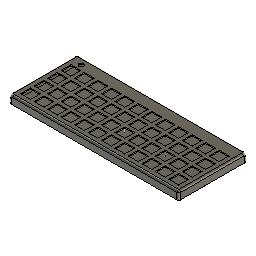
liteboard (Autodesk Fusion 360 design; units mm, degrees)
part number: 2026-04-12-12-30-01-683
Autodesk Fusion 360 part; units mm, degrees
(part 1 of 18)
sketch "草图2" plane through (0, 0, 0) normal (0, 0, 1) x (1, 0, 0)
  line L0 (4.2648, 0.88) -> (3.8878, 1.2675)
  line L1 (-10.3353, 1.2675) -> (0.4381, 1.2675)
  line L2 (0.0611, 0.88) -> (-0.1551, 0.3845)
  line L3 (0.4381, 1.2675) -> (0.0611, 0.88)
  line L4 (222.6289, -88.1864) -> (-10.3353, -88.1864)
  line L5 (-10.3353, -88.1864) -> (-10.3353, 1.2675)
  line L6 (222.6289, 1.2675) -> (222.6289, -88.1864)
  line L7 (4.5085, -0.1553) -> (4.481, 0.3845)
  line L8 (0.3176, -1.0941) -> (0.7811, -1.3723)
  line L9 (4.481, 0.3845) -> (4.2648, 0.88)
  line L10 (-0.1826, -0.1553) -> (-0.018, -0.6703)
  line L11 (3.8878, 1.2675) -> (222.6289, 1.2675)
  line L12 (4.0083, -1.0941) -> (4.3439, -0.6703)
  line L13 (3.0129, -1.4692) -> (3.5448, -1.3723)
  line L14 (4.3439, -0.6703) -> (4.5085, -0.1553)
  line L15 (0.7811, -1.3723) -> (1.3129, -1.4692)
  line L16 (-0.018, -0.6703) -> (0.3176, -1.0941)
  line L17 (3.5448, -1.3723) -> (4.0083, -1.0941)
  line L18 (-0.1551, 0.3845) -> (-0.1826, -0.1553)
  line L19 (1.3129, -1.4692) -> (3.0129, -1.4692)
  line L20 (-4.3556, -1.7588) -> (-4.8371, -1.663)
  line L21 (-5.9994, -3.4026) -> (-5.7267, -3.8108)
  line L22 (-3.6747, -3.4026) -> (-3.5789, -2.9211)
  line L23 (-3.9474, -2.0315) -> (-4.3556, -1.7588)
  line L24 (-4.8371, -4.1793) -> (-4.3556, -4.0835)
  line L25 (-5.7267, -3.8108) -> (-5.3185, -4.0835)
  line L26 (-4.8371, -1.663) -> (-5.3185, -1.7588)
  line L27 (-3.6747, -2.4397) -> (-3.9474, -2.0315)
  line L28 (-4.3556, -4.0835) -> (-3.9474, -3.8108)
  line L29 (-5.3185, -4.0835) -> (-4.8371, -4.1793)
  line L30 (-5.9994, -2.4397) -> (-6.0952, -2.9211)
  line L31 (-3.9474, -3.8108) -> (-3.6747, -3.4026)
  line L32 (-6.0952, -2.9211) -> (-5.9994, -3.4026)
  line L33 (-5.7267, -2.0315) -> (-5.9994, -2.4397)
  line L34 (-5.3185, -1.7588) -> (-5.7267, -2.0315)
  line L35 (-3.5789, -2.9211) -> (-3.6747, -2.4397)
  line L36 (-5.7267, -7.1115) -> (-5.9994, -7.5197)
  line L37 (-5.9994, -8.4826) -> (-5.7267, -8.8908)
  line L38 (-5.9994, -7.5197) -> (-6.0952, -8.0011)
  line L39 (-6.0952, -8.0011) -> (-5.9994, -8.4826)
  line L40 (-3.6747, -7.5197) -> (-3.9474, -7.1115)
  line L41 (-5.3185, -9.1635) -> (-4.8371, -9.2593)
  line L42 (-3.9474, -8.8908) -> (-3.6747, -8.4826)
  line L43 (-4.8371, -9.2593) -> (-4.3556, -9.1635)
  line L44 (-3.9474, -7.1115) -> (-4.3556, -6.8388)
  line L45 (-4.3556, -6.8388) -> (-4.8371, -6.743)
  line L46 (-4.8371, -6.743) -> (-5.3185, -6.8388)
  line L47 (-5.7267, -8.8908) -> (-5.3185, -9.1635)
  line L48 (-3.6747, -8.4826) -> (-3.5789, -8.0011)
  line L49 (-4.3556, -9.1635) -> (-3.9474, -8.8908)
  line L50 (-5.3185, -6.8388) -> (-5.7267, -7.1115)
  line L51 (-3.5789, -8.0011) -> (-3.6747, -7.5197)
  line L52 (2.8261, -21.8809) -> (3.418, -21.4267)
  line L53 (-1.3638, -20.1454) -> (-1.0782, -20.8347)
  line L54 (-1.0782, -17.9766) -> (-1.3638, -18.6659)
  line L55 (-0.0321, -21.8809) -> (0.6573, -22.1664)
  line L56 (4.1578, -18.6659) -> (3.8722, -17.9766)
  line L57 (2.8261, -16.9304) -> (2.1367, -16.6449)
  line L58 (-1.4611, -19.4056) -> (-1.3638, -20.1454)
  line L59 (3.8722, -17.9766) -> (3.418, -17.3846)
  line L60 (0.6573, -16.6449) -> (-0.0321, -16.9304)
  line L61 (2.1367, -16.6449) -> (1.397, -16.5475)
  line L62 (1.397, -16.5475) -> (0.6573, -16.6449)
  line L63 (3.418, -17.3846) -> (2.8261, -16.9304)
  line L64 (0.6573, -22.1664) -> (1.397, -22.2638)
  line L65 (3.8722, -20.8347) -> (4.1578, -20.1454)
  line L66 (-0.624, -21.4267) -> (-0.0321, -21.8809)
  line L67 (-0.624, -17.3846) -> (-1.0782, -17.9766)
  line L68 (1.397, -22.2638) -> (2.1367, -22.1664)
  line L69 (4.1578, -20.1454) -> (4.2551, -19.4056)
  line L70 (-0.0321, -16.9304) -> (-0.624, -17.3846)
  line L71 (4.2551, -19.4056) -> (4.1578, -18.6659)
  line L72 (2.1367, -22.1664) -> (2.8261, -21.8809)
  line L73 (3.418, -21.4267) -> (3.8722, -20.8347)
  line L74 (-1.0782, -20.8347) -> (-0.624, -21.4267)
  line L75 (-1.3638, -18.6659) -> (-1.4611, -19.4056)
  line L76 (-1.4611, -76.5812) -> (-1.3638, -77.3209)
  line L77 (0.6573, -73.8204) -> (-0.0321, -74.1059)
  line L78 (-1.0782, -75.1521) -> (-1.3638, -75.8414)
  line L79 (3.418, -74.5601) -> (2.8261, -74.1059)
  line L80 (0.6573, -79.3419) -> (1.397, -79.4393)
  line L81 (-0.0321, -79.0564) -> (0.6573, -79.3419)
  line L82 (3.8722, -75.1521) -> (3.418, -74.5601)
  line L83 (-0.624, -78.6022) -> (-0.0321, -79.0564)
  line L84 (3.418, -78.6022) -> (3.8722, -78.0102)
  line L85 (4.1578, -77.3209) -> (4.2551, -76.5812)
  line L86 (-1.3638, -75.8414) -> (-1.4611, -76.5812)
  line L87 (2.8261, -79.0564) -> (3.418, -78.6022)
  line L88 (2.1367, -73.8204) -> (1.397, -73.723)
  line L89 (1.397, -73.723) -> (0.6573, -73.8204)
  line L90 (1.397, -79.4393) -> (2.1367, -79.3419)
  line L91 (2.1367, -79.3419) -> (2.8261, -79.0564)
  line L92 (4.2551, -76.5812) -> (4.1578, -75.8414)
  line L93 (2.8261, -74.1059) -> (2.1367, -73.8204)
  line L94 (-0.624, -74.5601) -> (-1.0782, -75.1521)
  line L95 (-0.0321, -74.1059) -> (-0.624, -74.5601)
  line L96 (4.1578, -75.8414) -> (3.8722, -75.1521)
  line L97 (3.8722, -78.0102) -> (4.1578, -77.3209)
  line L98 (-1.3638, -77.3209) -> (-1.0782, -78.0102)
  line L99 (-1.0782, -78.0102) -> (-0.624, -78.6022)
  line L100 (-0.0321, -35.9805) -> (-0.624, -36.4347)
  line L101 (-0.624, -40.4767) -> (-0.0321, -40.9309)
  line L102 (2.1367, -35.6949) -> (1.397, -35.5975)
  line L103 (3.8722, -37.0266) -> (3.418, -36.4347)
  line L104 (4.1578, -39.1954) -> (4.2551, -38.4557)
  line L105 (-0.624, -36.4347) -> (-1.0782, -37.0266)
  line L106 (1.397, -41.3138) -> (2.1367, -41.2164)
  line L107 (-1.0782, -37.0266) -> (-1.3638, -37.7159)
  line L108 (3.8722, -39.8847) -> (4.1578, -39.1954)
  line L109 (-1.3638, -37.7159) -> (-1.4611, -38.4557)
  line L110 (1.397, -35.5975) -> (0.6573, -35.6949)
  line L111 (-1.3638, -39.1954) -> (-1.0782, -39.8847)
  line L112 (-1.4611, -38.4557) -> (-1.3638, -39.1954)
  line L113 (2.8261, -40.9309) -> (3.418, -40.4767)
  line L114 (-1.0782, -39.8847) -> (-0.624, -40.4767)
  line L115 (0.6573, -35.6949) -> (-0.0321, -35.9805)
  line L116 (4.2551, -38.4557) -> (4.1578, -37.7159)
  line L117 (3.418, -40.4767) -> (3.8722, -39.8847)
  line L118 (3.418, -36.4347) -> (2.8261, -35.9805)
  line L119 (2.1367, -41.2164) -> (2.8261, -40.9309)
  line L120 (2.8261, -35.9805) -> (2.1367, -35.6949)
  line L121 (4.1578, -37.7159) -> (3.8722, -37.0266)
  line L122 (-0.0321, -40.9309) -> (0.6573, -41.2164)
  line L123 (0.6573, -41.2164) -> (1.397, -41.3138)
  line L124 (-0.624, -55.4974) -> (-1.0782, -56.0893)
  line L125 (0.6573, -54.7577) -> (-0.0321, -55.0432)
  line L126 (2.8261, -59.9936) -> (3.418, -59.5394)
  line L127 (2.1367, -54.7577) -> (1.397, -54.6603)
  line L128 (3.418, -59.5394) -> (3.8722, -58.9475)
  line L129 (3.8722, -58.9475) -> (4.1578, -58.2582)
  line L130 (-1.3638, -56.7787) -> (-1.4611, -57.5184)
  line L131 (4.1578, -58.2582) -> (4.2551, -57.5184)
  line L132 (-0.0321, -55.0432) -> (-0.624, -55.4974)
  line L133 (4.1578, -56.7787) -> (3.8722, -56.0893)
  line L134 (-1.4611, -57.5184) -> (-1.3638, -58.2582)
  line L135 (-0.624, -59.5394) -> (-0.0321, -59.9936)
  line L136 (-1.0782, -56.0893) -> (-1.3638, -56.7787)
  line L137 (0.6573, -60.2792) -> (1.397, -60.3766)
  line L138 (1.397, -60.3766) -> (2.1367, -60.2792)
  line L139 (-1.3638, -58.2582) -> (-1.0782, -58.9475)
  line L140 (1.397, -54.6603) -> (0.6573, -54.7577)
  line L141 (3.418, -55.4974) -> (2.8261, -55.0432)
  line L142 (2.1367, -60.2792) -> (2.8261, -59.9936)
  line L143 (-0.0321, -59.9936) -> (0.6573, -60.2792)
  line L144 (4.2551, -57.5184) -> (4.1578, -56.7787)
  line L145 (3.8722, -56.0893) -> (3.418, -55.4974)
  line L146 (-1.0782, -58.9475) -> (-0.624, -59.5394)
  line L147 (2.8261, -55.0432) -> (2.1367, -54.7577)
  line L148 (175.0892, -23.1507) -> (175.1842, -23.6313)
  line L149 (200.443, -3.4264) -> (200.5548, -3.1425)
  line L150 (195.6981, -2.3541) -> (195.408, -2.2378)
  line L151 (206.2125, -2.532) -> (206.1424, -2.2351)
  line L152 (19.9512, -10.5182) -> (19.879, -10.5602)
  line L153 (172.2522, -5.3569) -> (167.1323, -5.3569)
  line L154 (1.3129, -12.4692) -> (2.985, -12.4692)
  line L155 (190.9024, 0.21) -> (190.8125, 0.6041)
  line L156 (172.2256, -3.3861) -> (172.2242, -3.418)
  line L157 (9.181, -1.759) -> (8.7706, -2.0343)
  line L158 (195.408, -2.2378) -> (195.0968, -2.2673)
  line L159 (167.1323, -5.3569) -> (166.9467, -5.3938)
  line L160 (215.5423, -1.3966) -> (215.5423, -11.302)
  line L161 (196.5703, -6.8777) -> (194.9024, -6.8777)
  line L162 (10.1501, -1.7611) -> (9.6657, -1.663)
  line L163 (173.5966, -1.369) -> (173.3141, -1.4382)
  line L164 (2.985, -12.4692) -> (3.1779, -12.6621)
  line L165 (176.3444, -21.8935) -> (175.864, -21.99)
  line L166 (215.6027, -11.9249) -> (215.8415, -12.1417)
  line L167 (8.7706, -2.0343) -> (8.4979, -2.4465)
  line L168 (190.9024, -0.5069) -> (190.9024, 0.21)
  line L169 (197.593, 0.2231) -> (191.8334, 0.2231)
  line L170 (201.9182, -1.8376) -> (202.224, -1.9247)
  line L171 (156.1344, -61.7447) -> (156.4058, -62.1522)
  line L172 (198.2393, 0.2231) -> (198.1398, 0.2231)
  line L173 (0.7971, -12.3782) -> (1.3129, -12.4692)
  line L174 (194.8338, -3.3523) -> (195.0969, -3.521)
  line L175 (10.8239, -8.4863) -> (164.9732, -8.4863)
  line L176 (156.4056, -24.0392) -> (156.8122, -24.3125)
  line L177 (180.5338, -0.9789) -> (180.7794, -1.2929)
  line L178 (167.3333, -6.3272) -> (189.3463, -6.3272)
  line L179 (189.3011, -6.8777) -> (167.1355, -6.8777)
  line L180 (201.5865, -1.3167) -> (201.688, -1.6181)
  line L181 (172.9618, -2.1747) -> (173.0851, -2.4381)
  line L182 (4.0055, -41.3139) -> (3.7341, -41.7214)
  line L183 (3.6389, -42.2017) -> (3.7341, -42.6819)
  line L184 (164.2644, -9.5479) -> (18.415, -9.5479)
  line L185 (175.3144, -1.5898) -> (175.5226, -1.8185)
  line L186 (197.8695, -1.6165) -> (198.0055, -1.3392)
  line L187 (10.5503, -8.8932) -> (10.8239, -8.4863)
  line L188 (182.2626, 0.21) -> (182.1727, 0.6041)
  line L189 (201.168, -0.6121) -> (202.1153, -0.6121)
  line L190 (202.224, -1.9247) -> (203.1744, -2.8751)
  line L191 (202.8355, -0.9556) -> (202.6463, -0.7323)
  line L192 (4.0074, -22.262) -> (3.7349, -22.6694)
  line L193 (195.9027, -2.5903) -> (195.6981, -2.3541)
  line L194 (10.1419, -6.8377) -> (9.6608, -6.743)
  line L195 (176.3475, -0.7849) -> (176.0783, -0.6326)
  line L196 (172.2299, -3.3545) -> (172.2256, -3.3861)
  line L197 (156.4058, -60.3767) -> (156.1344, -60.7842)
  line L198 (199.2895, -0.5484) -> (199.3507, -0.1912)
  line L199 (156.0392, -61.2644) -> (156.1344, -61.7447)
  line L200 (216.1544, -12.2202) -> (216.4673, -12.1417)
  line L201 (0.3435, -12.1163) -> (0.7971, -12.3782)
  line L202 (190.7902, -3.3527) -> (194.8338, -3.3523)
  line L203 (190.8739, -3.5643) -> (190.7902, -3.3527)
  line L204 (4.8954, -21.8935) -> (4.4148, -21.9896)
  line L205 (198.1922, -0.9586) -> (198.3525, -0.832)
  line L206 (201.637, -1.0027) -> (201.5865, -1.3167)
  line L207 (172.2313, -5.2888) -> (172.2522, -5.3569)
  line L208 (202.6463, -0.7323) -> (202.3795, -0.6121)
  line L209 (8.5005, -8.4821) -> (8.7726, -8.89)
  line L210 (198.7028, -0.925) -> (199.0496, -0.8201)
  line L211 (194.2339, -79.8483) -> (194.1393, -80.3294)
  line L212 (10.5503, -7.1091) -> (10.1419, -6.8377)
  line L213 (205.9467, -3.063) -> (206.1424, -2.8289)
  line L214 (18.2294, -9.5848) -> (18.072, -9.69)
  line L215 (190.8695, -5.1322) -> (190.9024, -4.8901)
  line L216 (166.9498, -6.9146) -> (166.7925, -7.0198)
  line L217 (182.1751, -0.9789) -> (182.2626, -0.59)
  line L218 (199.8039, -2.3916) -> (199.52, -2.5034)
  line L219 (216.7666, -11.302) -> (216.7666, -1.143)
  line L220 (202.9101, -1.2386) -> (202.8355, -0.9556)
  line L221 (205.3623, -1.8958) -> (205.0973, -2.0469)
  line L222 (180.5363, 0.6041) -> (180.4463, 0.21)
  line L223 (205.3623, -3.1682) -> (205.667, -3.1846)
  line L224 (190.5605, 0.92) -> (190.1964, 1.0954)
  line L225 (203.3317, -2.9802) -> (203.5174, -3.0171)
  line L226 (178.803, -0.8218) -> (178.6173, -0.7849)
  line L227 (199.52, -2.5034) -> (199.3163, -2.7304)
  line L228 (3.521, -12.8042) -> (16.129, -12.8042)
  line L229 (205.0973, -3.0171) -> (205.3623, -3.1682)
  line L230 (9.6608, -9.2593) -> (10.1419, -9.1646)
  line L231 (6.0579, -22.6665) -> (5.7844, -22.2598)
  line L232 (194.3243, -4.9814) -> (194.0618, -4.9249)
  line L233 (215.5423, -11.302) -> (215.4944, -11.621)
  line L234 (15.9281, -11.8339) -> (4.2428, -11.8339)
  line L235 (178.9604, -0.927) -> (178.803, -0.8218)
  line L236 (205.667, -1.8794) -> (205.3623, -1.8958)
  line L237 (189.0861, 0.21) -> (189.0861, -0.59)
  line L238 (9.2008, -4.0913) -> (9.6871, -4.179)
  line L239 (0.7971, -9.5438) -> (0.3435, -9.8057)
  line L240 (8.7726, -7.1123) -> (8.5005, -7.5202)
  line L241 (164.7723, -7.516) -> (10.8239, -7.516)
  line L242 (173.8815, -1.4273) -> (173.5966, -1.369)
  line L243 (8.7726, -8.89) -> (9.18, -9.1629)
  line L244 (216.5873, -0.7102) -> (215.4443, 0.4328)
  line L245 (189.3463, -6.3272) -> (189.2636, -6.5975)
  line L246 (205.0973, -2.0469) -> (203.7184, -2.0469)
  line L247 (197.6227, -1.8022) -> (197.8695, -1.6165)
  line L248 (194.6816, -5.3671) -> (194.5428, -5.1373)
  line L249 (4.4148, -21.9896) -> (4.0074, -22.262)
  line L250 (166.7925, -7.0198) -> (164.2644, -9.5479)
  line L251 (165.3162, -8.3442) -> (167.3333, -6.3272)
  line L252 (175.8118, -1.9279) -> (174.3183, -1.9279)
  line L253 (173.3141, -1.4382) -> (173.0884, -1.6216)
  line L254 (199.0496, -0.8201) -> (199.2895, -0.5484)
  line L255 (15.9233, -3.3705) -> (15.9425, -3.3693)
  line L256 (199.2357, -3.0246) -> (198.4743, -3.786)
  line L257 (19.8151, -10.6139) -> (7.7625, -22.6665)
  line L258 (181.5565, 1.0954) -> (181.1524, 1.0954)
  line L259 (4.5116, -10.7923) -> (4.3529, -10.2689)
  line L260 (180.4463, -0.59) -> (180.5338, -0.9789)
  line L261 (198.001, -1.0303) -> (198.1922, -0.9586)
  line L262 (200.5276, -2.8386) -> (200.3673, -2.5791)
  line L263 (190.8125, 0.6041) -> (190.5605, 0.92)
  line L264 (164.9732, -8.4863) -> (165.1589, -8.4494)
  line L265 (156.8122, -41.0408) -> (156.4058, -41.3139)
  line L266 (202.3795, -0.6121) -> (214.7579, -0.6121)
  line L267 (181.9295, -1.2929) -> (182.1751, -0.9789)
  line L268 (15.9041, -3.3709) -> (15.9233, -3.3705)
  line L269 (10.8381, -3.3709) -> (15.9041, -3.3709)
  line L270 (200.9144, 0.6121) -> (200.6801, 0.5655)
  line L271 (198.1618, -6.6507) -> (197.9434, -6.6507)
  line L272 (8.4979, -2.4465) -> (8.405, -2.9318)
  line L273 (175.5226, -1.8185) -> (175.8118, -1.9279)
  line L274 (193.7985, -4.9771) -> (193.5774, -5.1294)
  line L275 (181.1524, 1.0954) -> (180.7882, 0.92)
  line L276 (4.4119, -24.3125) -> (4.4119, -41.0408)
  line L277 (198.3322, -4.129) -> (198.3322, -6.0986)
  line L278 (197.6871, -6.4844) -> (197.3834, -6.4506)
  line L279 (3.6389, -23.1501) -> (3.7337, -23.6309)
  line L280 (215.8415, -12.1417) -> (216.1544, -12.2202)
  line L281 (189.1761, 0.6041) -> (189.0861, 0.21)
  line L282 (176.8251, -21.9878) -> (176.3444, -21.8935)
  line L283 (3.7349, -22.6694) -> (3.6389, -23.1501)
  line L284 (189.7922, 1.0954) -> (189.4281, 0.92)
  line L285 (9.6657, -1.663) -> (9.181, -1.759)
  line L286 (177.5102, -60.7842) -> (177.2389, -60.3767)
  line L287 (-0.1723, -10.6991) -> (-0.1723, -11.2229)
  line L288 (175.864, -21.99) -> (175.457, -22.2627)
  line L289 (190.1964, 1.0954) -> (189.7922, 1.0954)
  line L290 (171.9053, -13.3122) -> (185.5007, -13.3122)
  line L291 (189.1736, -0.9789) -> (189.4193, -1.2929)
  line L292 (215.0114, 0.6121) -> (200.9144, 0.6121)
  line L293 (158.4602, -60.7842) -> (158.1888, -60.3767)
  line L294 (216.8145, -11.621) -> (216.7666, -11.302)
  line L295 (195.8825, -60.1036) -> (195.8825, -43.3625)
  line L296 (194.2345, -42.6819) -> (194.5059, -43.0894)
  line L297 (201.3539, -9.7544) -> (201.0692, -9.8528)
  line L298 (200.2237, -9.1925) -> (199.9543, -9.3449)
  line L299 (177.2389, -41.3139) -> (176.8325, -41.0408)
  line L300 (209.4715, -9.0376) -> (209.6395, -9.2629)
  line L301 (175.8664, -81.4897) -> (176.3474, -81.5853)
  line L302 (205.1665, -11.5952) -> (204.8563, -11.7579)
  line L303 (175.1845, -60.7842) -> (175.0892, -61.2644)
  line L304 (209.9181, -10.4074) -> (210.2759, -10.3948)
  line L305 (203.0941, -11.1739) -> (203.07, -10.8729)
  line L306 (199.3025, -4.33) -> (199.9218, -3.7107)
  line L307 (194.2345, -61.7447) -> (194.5059, -62.1522)
  line L308 (202.915, -10.6139) -> (202.6612, -10.4504)
  line L309 (202.3612, -10.4164) -> (202.0772, -10.5189)
  line L310 (201.7756, -6.3295) -> (201.8474, -6.6507)
  line L311 (199.4729, -6.6507) -> (199.451, -6.3551)
  line L312 (199.9218, -3.7107) -> (200.216, -3.6301)
  line L313 (167.9834, -17.2341) -> (171.9053, -13.3122)
  line L314 (196.6555, -61.2644) -> (196.5603, -60.7842)
  line L315 (175.8622, -79.1663) -> (175.4553, -79.4399)
  line L316 (199.1561, -8.4813) -> (198.9102, -8.5383)
  line L317 (196.5608, -79.8483) -> (196.2894, -79.4399)
  line L318 (156.407, -22.2627) -> (156.1349, -22.6702)
  line L319 (163.5579, -16.4059) -> (163.3723, -16.4428)
  line L320 (163.2149, -16.548) -> (157.7751, -21.9878)
  line L321 (201.0073, -9.5495) -> (200.8146, -9.3074)
  line L322 (200.5329, -9.1791) -> (200.2237, -9.1925)
  line L323 (200.8146, -9.3074) -> (200.5329, -9.1791)
  line L324 (194.9123, -62.4253) -> (194.9123, -79.1663)
  line L325 (201.8474, -6.6507) -> (199.4729, -6.6507)
  line L326 (207.5885, -14.8215) -> (207.8381, -14.6519)
  line L327 (199.9543, -9.3449) -> (199.8121, -9.3449)
  line L328 (177.5102, -61.7447) -> (177.6055, -61.2644)
  line L329 (157.2943, -21.8935) -> (156.814, -21.99)
  line L330 (156.1342, -23.6313) -> (156.4056, -24.0392)
  line L331 (156.814, -21.99) -> (156.407, -22.2627)
  line L332 (156.1349, -22.6702) -> (156.0392, -23.1507)
  line L333 (158.5555, -80.3294) -> (158.4608, -79.8483)
  line L334 (158.1862, -81.2176) -> (158.459, -80.8102)
  line L335 (199.8121, -9.3449) -> (199.8414, -9.0942)
  line L336 (207.1491, -12.8136) -> (206.802, -12.8325)
  line L337 (199.3025, -6.0986) -> (199.3025, -4.33)
  line L338 (195.8825, -62.4253) -> (196.2889, -62.1522)
  line L339 (206.7888, -14.5552) -> (207.0032, -14.7675)
  line L340 (177.5102, -41.7214) -> (177.2389, -41.3139)
  line L341 (209.4835, -8.063) -> (209.6394, -8.263)
  line L342 (158.1894, -79.4399) -> (157.7825, -79.1663)
  line L343 (196.5591, -80.8102) -> (196.6555, -80.3294)
  line L344 (194.9123, -41.0408) -> (194.5059, -41.3139)
  line L345 (205.9605, -12.1223) -> (205.808, -11.807)
  line L346 (198.9102, -8.5383) -> (198.8429, -8.2682)
  line L347 (204.8563, -11.7579) -> (204.3641, -11.7579)
  line L348 (176.8325, -41.0408) -> (176.8325, -24.3125)
  line L349 (205.5162, -11.6133) -> (205.1665, -11.5952)
  line L350 (207.4581, -12.9728) -> (207.1491, -12.8136)
  line L351 (206.2819, -12.1114) -> (205.9605, -12.1223)
  line L352 (196.6555, -42.2017) -> (196.5603, -41.7214)
  line L353 (209.6059, -10.232) -> (209.9181, -10.4074)
  line L354 (212.2314, -10.4073) -> (212.5433, -10.2319)
  line L355 (199.7749, -8.8507) -> (199.6222, -8.6497)
  line L356 (177.2394, -79.4399) -> (176.8325, -79.1663)
  line L357 (157.7783, -81.4897) -> (158.1862, -81.2176)
  line L358 (194.9123, -79.1663) -> (194.5053, -79.4399)
  line L359 (196.2894, -79.4399) -> (195.8825, -79.1663)
  line L360 (195.8825, -41.0408) -> (195.8825, -24.3125)
  line L361 (209.4304, -9.9199) -> (209.6059, -10.232)
  line L362 (158.459, -80.8102) -> (158.5555, -80.3294)
  line L363 (156.8164, -81.4897) -> (157.2973, -81.5853)
  line L364 (194.9123, -43.3625) -> (194.9123, -60.1036)
  line L365 (196.5499, -22.647) -> (204.6418, -14.5552)
  line L366 (199.4054, -8.5203) -> (199.1561, -8.4813)
  line L367 (194.9123, -60.1036) -> (194.5059, -60.3767)
  line L368 (199.8414, -9.0942) -> (199.7749, -8.8507)
  line L369 (176.8283, -81.4897) -> (177.2362, -81.2176)
  line L370 (199.6222, -8.6497) -> (199.4054, -8.5203)
  line L371 (196.5603, -60.7842) -> (196.2889, -60.3767)
  line L372 (196.5653, -23.6196) -> (196.6554, -23.1318)
  line L373 (194.9123, -24.3125) -> (194.9123, -41.0408)
  line L374 (212.6779, -8.4885) -> (212.5099, -8.2631)
  line L375 (202.056, -10.2184) -> (201.9041, -9.9582)
  line L376 (157.7751, -21.9878) -> (157.2943, -21.8935)
  line L377 (175.8622, -43.3625) -> (175.8622, -60.1036)
  line L378 (167.4394, -16.4059) -> (163.5579, -16.4059)
  line L379 (199.451, -6.3551) -> (199.3025, -6.0986)
  line L380 (156.0392, -23.1507) -> (156.1342, -23.6313)
  line L381 (156.0392, -42.2017) -> (156.1344, -42.6819)
  line L382 (196.2889, -62.1522) -> (196.5603, -61.7447)
  line L383 (156.4058, -41.3139) -> (156.1344, -41.7214)
  line L384 (204.6418, -14.5552) -> (206.7888, -14.5552)
  line L385 (194.1393, -80.3294) -> (194.2357, -80.8102)
  line L386 (175.0892, -42.2017) -> (175.1845, -42.6819)
  line L387 (175.1845, -42.6819) -> (175.4558, -43.0894)
  line L388 (175.4558, -43.0894) -> (175.8622, -43.3625)
  line L389 (175.4558, -41.3139) -> (175.1845, -41.7214)
  line L390 (176.8325, -62.4253) -> (177.2389, -62.1522)
  line L391 (194.5059, -62.1522) -> (194.9123, -62.4253)
  line L392 (194.2315, -23.6245) -> (194.5031, -24.0366)
  line L393 (204.3489, -11.4872) -> (204.2266, -11.2452)
  line L394 (212.7375, -8.7631) -> (212.6779, -8.4885)
  line L395 (196.2862, -81.2176) -> (196.5591, -80.8102)
  line L396 (205.808, -11.807) -> (205.5162, -11.6133)
  line L397 (175.1856, -80.8102) -> (175.4585, -81.2176)
  line L398 (204.3641, -11.7579) -> (204.3489, -11.4872)
  line L399 (204.2266, -11.2452) -> (204.0177, -11.0724)
  line L400 (175.8622, -41.0408) -> (175.4558, -41.3139)
  line L401 (198.4239, -7.9208) -> (198.4014, -7.7372)
  line L402 (201.6528, -9.7922) -> (201.3539, -9.7544)
  line L403 (195.8825, -43.3625) -> (196.2889, -43.0894)
  line L404 (196.6554, -23.1318) -> (196.5499, -22.647)
  line L405 (194.5059, -41.3139) -> (194.2345, -41.7214)
  line L406 (212.5099, -8.2631) -> (212.6658, -8.0631)
  line L407 (157.7825, -62.4253) -> (158.1888, -62.1522)
  line L408 (158.4602, -61.7447) -> (158.5555, -61.2644)
  line L409 (208.0035, -14.0879) -> (207.8851, -13.8103)
  line L410 (185.5007, -13.3122) -> (176.8251, -21.9878)
  line L411 (167.6403, -17.3762) -> (167.826, -17.3392)
  line L412 (139.1388, -62.1522) -> (139.4102, -61.7447)
  line L413 (156.8122, -24.3125) -> (156.8122, -41.0408)
  line L414 (138.7324, -79.1663) -> (138.7324, -62.4253)
  line L415 (167.826, -17.3392) -> (167.9834, -17.2341)
  line L416 (163.7589, -17.3762) -> (167.6403, -17.3762)
  line L417 (158.5555, -23.1536) -> (158.4612, -22.6739)
  line L418 (176.8325, -79.1663) -> (176.8325, -62.4253)
  line L419 (158.4597, -23.6331) -> (158.5555, -23.1536)
  line L420 (203.757, -10.9977) -> (203.4883, -11.0335)
  line L421 (175.8622, -62.4253) -> (175.8622, -79.1663)
  line L422 (206.5706, -12.253) -> (206.2819, -12.1114)
  line L423 (158.4612, -22.6739) -> (163.7589, -17.3762)
  line L424 (194.1392, -42.2017) -> (194.2345, -42.6819)
  line L425 (195.8825, -24.3125) -> (196.2936, -24.0347)
  line L426 (209.4119, -8.763) -> (209.4715, -9.0376)
  line L427 (196.2889, -60.3767) -> (195.8825, -60.1036)
  line L428 (138.7324, -43.3625) -> (139.1388, -43.0894)
  line L429 (139.5054, -61.2644) -> (139.4102, -60.7842)
  line L430 (139.1388, -60.3767) -> (138.7324, -60.1036)
  line L431 (194.2357, -80.8102) -> (194.5086, -81.2176)
  line L432 (194.1393, -23.1397) -> (194.2315, -23.6245)
  line L433 (212.6779, -9.0378) -> (212.7375, -8.7631)
  line L434 (176.8325, -24.3125) -> (177.2384, -24.0399)
  line L435 (175.4585, -81.2176) -> (175.8664, -81.4897)
  line L436 (196.2889, -43.0894) -> (196.5603, -42.6819)
  line L437 (209.4415, -7.567) -> (209.4142, -7.8191)
  line L438 (201.9041, -9.9582) -> (201.6528, -9.7922)
  line L439 (175.0892, -80.3294) -> (175.1856, -80.8102)
  line L440 (138.7324, -41.0408) -> (138.7324, -24.3125)
  line L441 (139.4102, -42.6819) -> (139.5054, -42.2017)
  line L442 (194.52, -22.2499) -> (194.2407, -22.6568)
  line L443 (212.7078, -7.567) -> (213.089, -7.567)
  line L444 (177.2384, -24.0399) -> (177.5097, -23.6331)
  line L445 (177.6055, -23.1536) -> (177.5112, -22.6739)
  line L446 (196.2889, -41.3139) -> (195.8825, -41.0408)
  line L447 (145.7248, -16.3602) -> (167.4851, -16.3602)
  line L448 (139.1383, -24.0399) -> (139.4096, -23.6331)
  line L449 (139.5054, -23.1536) -> (139.4112, -22.6739)
  line L450 (177.2389, -60.3767) -> (176.8325, -60.1036)
  line L451 (177.6055, -42.2017) -> (177.5102, -41.7214)
  line L452 (157.2973, -81.5853) -> (157.7783, -81.4897)
  line L453 (177.2362, -81.2176) -> (177.5091, -80.8102)
  line L454 (156.0392, -80.3294) -> (156.1356, -80.8102)
  line L455 (156.4085, -81.2176) -> (156.8164, -81.4897)
  line L456 (203.4883, -11.0335) -> (203.2563, -11.1739)
  line L457 (194.5031, -24.0366) -> (194.9123, -24.3125)
  line L458 (194.5059, -60.3767) -> (194.2345, -60.7842)
  line L459 (212.7351, -7.8191) -> (212.7078, -7.567)
  line L460 (206.802, -12.8325) -> (206.7587, -12.5138)
  line L461 (204.0177, -11.0724) -> (203.757, -10.9977)
  line L462 (175.1845, -61.7447) -> (175.4558, -62.1522)
  line L463 (212.7187, -9.9199) -> (212.7063, -9.5623)
  line L464 (194.5059, -43.0894) -> (194.9123, -43.3625)
  line L465 (210.2759, -10.3948) -> (210.575, -10.1979)
  line L466 (196.5603, -61.7447) -> (196.6555, -61.2644)
  line L467 (177.5112, -22.6739) -> (186.1109, -14.0742)
  line L468 (195.4199, -21.8937) -> (194.9343, -21.9818)
  line L469 (139.4102, -41.7214) -> (139.1388, -41.3139)
  line L470 (176.8325, -60.1036) -> (176.8325, -43.3625)
  line L471 (194.9343, -21.9818) -> (194.52, -22.2499)
  line L472 (211.5746, -10.1985) -> (211.8737, -10.3949)
  line L473 (207.8851, -13.8103) -> (207.6559, -13.614)
  line L474 (177.6055, -61.2644) -> (177.5102, -60.7842)
  line L475 (158.5555, -42.2017) -> (158.4602, -41.7214)
  line L476 (139.4096, -23.6331) -> (139.5054, -23.1536)
  line L477 (139.1388, -41.3139) -> (138.7324, -41.0408)
  line L478 (138.7324, -24.3125) -> (139.1383, -24.0399)
  line L479 (158.1888, -43.0894) -> (158.4602, -42.6819)
  line L480 (158.1888, -41.3139) -> (157.7825, -41.0408)
  line L481 (177.6055, -80.3294) -> (177.5108, -79.8483)
  line L482 (156.1356, -80.8102) -> (156.4085, -81.2176)
  line L483 (158.4602, -42.6819) -> (158.5555, -42.2017)
  line L484 (213.089, -7.567) -> (213.2632, -7.8436)
  line L485 (196.6555, -80.3294) -> (196.5608, -79.8483)
  line L486 (207.6559, -13.614) -> (207.6441, -13.2666)
  line L487 (211.3492, -10.3662) -> (211.5746, -10.1985)
  line L488 (207.6441, -13.2666) -> (207.4581, -12.9728)
  line L489 (156.1339, -79.8483) -> (156.0392, -80.3294)
  line L490 (198.6707, -8.0495) -> (198.4239, -7.9208)
  line L491 (195.8825, -79.1663) -> (195.8825, -62.4253)
  line L492 (201.0692, -9.8528) -> (201.0073, -9.5495)
  line L493 (139.4112, -22.6739) -> (145.7248, -16.3602)
  line L494 (177.5108, -79.8483) -> (177.2394, -79.4399)
  line L495 (167.4851, -16.3602) -> (167.4394, -16.4059)
  line L496 (138.7324, -60.1036) -> (138.7324, -43.3625)
  line L497 (139.1388, -43.0894) -> (139.4102, -42.6819)
  line L498 (177.2389, -43.0894) -> (177.5102, -42.6819)
  line L499 (139.5054, -42.2017) -> (139.4102, -41.7214)
  line L500 (156.8122, -79.1663) -> (156.4053, -79.4399)
  line L501 (157.7825, -41.0408) -> (157.7825, -24.3125)
  line L502 (158.4602, -41.7214) -> (158.1888, -41.3139)
  line L503 (177.2389, -62.1522) -> (177.5102, -61.7447)
  line L504 (157.7825, -60.1036) -> (157.7825, -43.3625)
  line L505 (177.5097, -23.6331) -> (177.6055, -23.1536)
  line L506 (138.7324, -62.4253) -> (139.1388, -62.1522)
  line L507 (139.4102, -61.7447) -> (139.5054, -61.2644)
  line L508 (195.902, -21.9991) -> (195.4199, -21.8937)
  line L509 (212.6658, -8.0631) -> (212.7351, -7.8191)
  line L510 (207.9867, -14.3892) -> (208.0035, -14.0879)
  line L511 (194.2407, -22.6568) -> (194.1393, -23.1397)
  line L512 (213.2632, -7.8436) -> (213.5483, -8.0034)
  line L513 (212.5099, -9.2631) -> (212.6779, -9.0378)
  line L514 (175.4553, -79.4399) -> (175.1839, -79.8483)
  line L515 (212.5433, -10.2319) -> (212.7187, -9.9199)
  line L516 (209.4714, -8.4883) -> (209.4119, -8.763)
  line L517 (209.6394, -8.263) -> (209.4714, -8.4883)
  line L518 (198.329, -7.567) -> (209.4415, -7.567)
  line L519 (198.4014, -7.7372) -> (198.329, -7.567)
  line L520 (194.1392, -61.2644) -> (194.2345, -61.7447)
  line L521 (203.827, -14.0742) -> (195.902, -21.9991)
  line L522 (3.3353, -12.7672) -> (3.521, -12.8042)
  line L523 (163.3723, -16.4428) -> (163.2149, -16.548)
  line L524 (207.2895, -14.8629) -> (207.5885, -14.8215)
  line L525 (209.4428, -9.5621) -> (209.4304, -9.9199)
  line L526 (211.8737, -10.3949) -> (212.2314, -10.4073)
  line L527 (196.5603, -41.7214) -> (196.2889, -41.3139)
  line L528 (194.2345, -41.7214) -> (194.1392, -42.2017)
  line L529 (175.457, -22.2627) -> (175.185, -22.6702)
  line L530 (202.6612, -10.4504) -> (202.3612, -10.4164)
  line L531 (175.1839, -79.8483) -> (175.0892, -80.3294)
  line L532 (202.415, -5.6873) -> (202.0993, -5.7801)
  line L533 (212.5142, -6.6507) -> (203.0295, -6.6507)
  line L534 (202.0772, -10.5189) -> (202.056, -10.2184)
  line L535 (209.4142, -7.8191) -> (209.4835, -8.063)
  line L536 (211.0747, -10.4256) -> (211.3492, -10.3662)
  line L537 (195.3974, -81.5853) -> (195.8783, -81.4897)
  line L538 (175.8622, -60.1036) -> (175.4558, -60.3767)
  line L539 (194.2345, -60.7842) -> (194.1392, -61.2644)
  line L540 (203.07, -10.8729) -> (202.915, -10.6139)
  line L541 (209.6395, -9.2629) -> (209.4428, -9.5621)
  line L542 (158.4608, -79.8483) -> (158.1894, -79.4399)
  line L543 (158.1888, -62.1522) -> (158.4602, -61.7447)
  line L544 (175.4558, -62.1522) -> (175.8622, -62.4253)
  line L545 (207.0032, -14.7675) -> (207.2895, -14.8629)
  line L546 (196.5603, -42.6819) -> (196.6555, -42.2017)
  line L547 (207.8381, -14.6519) -> (207.9867, -14.3892)
  line L548 (157.7825, -79.1663) -> (157.7825, -62.4253)
  line L549 (175.185, -22.6702) -> (175.0892, -23.1507)
  line L550 (175.1842, -23.6313) -> (175.4556, -24.0392)
  line L551 (175.8622, -24.3125) -> (175.8622, -41.0408)
  line L552 (156.8122, -60.1036) -> (156.4058, -60.3767)
  line L553 (214.1642, -7.8552) -> (214.3454, -7.5832)
  line L554 (156.4058, -43.0894) -> (156.8122, -43.3625)
  line L555 (214.1176, -6.4698) -> (214.101, -6.1558)
  line L556 (213.9877, -6.7562) -> (214.1176, -6.4698)
  line L557 (156.1344, -60.7842) -> (156.0392, -61.2644)
  line L558 (194.5053, -79.4399) -> (194.2339, -79.8483)
  line L559 (156.4058, -62.1522) -> (156.8122, -62.4253)
  line L560 (175.4556, -24.0392) -> (175.8622, -24.3125)
  line L561 (175.1845, -41.7214) -> (175.0892, -42.2017)
  line L562 (198.8429, -8.2682) -> (198.6707, -8.0495)
  line L563 (196.2936, -24.0347) -> (196.5653, -23.6196)
  line L564 (206.7587, -12.5138) -> (206.5706, -12.253)
  line L565 (186.1109, -14.0742) -> (203.827, -14.0742)
  line L566 (195.8783, -81.4897) -> (196.2862, -81.2176)
  line L567 (207.3526, -6.1337) -> (207.51, -6.0285)
  line L568 (212.7063, -9.5623) -> (212.5099, -9.2631)
  line L569 (176.3474, -81.5853) -> (176.8283, -81.4897)
  line L570 (203.2563, -11.1739) -> (203.0941, -11.1739)
  line L571 (210.8002, -10.3659) -> (211.0747, -10.4256)
  line L572 (175.4558, -60.3767) -> (175.1845, -60.7842)
  line L573 (194.5086, -81.2176) -> (194.9164, -81.4897)
  line L574 (194.9164, -81.4897) -> (195.3974, -81.5853)
  line L575 (158.5555, -61.2644) -> (158.4602, -60.7842)
  line L576 (157.7825, -43.3625) -> (158.1888, -43.0894)
  line L577 (210.575, -10.1979) -> (210.8002, -10.3659)
  line L578 (175.0892, -61.2644) -> (175.1845, -61.7447)
  line L579 (156.1344, -42.6819) -> (156.4058, -43.0894)
  line L580 (156.1344, -41.7214) -> (156.0392, -42.2017)
  line L581 (207.3173, -4.6354) -> (207.2367, -4.9296)
  line L582 (199.6558, -4.5177) -> (199.6877, -4.8097)
  line L583 (156.8122, -43.3625) -> (156.8122, -60.1036)
  line L584 (213.6754, -5.7176) -> (213.362, -5.6919)
  line L585 (208.444, -5.3314) -> (208.5558, -5.0475)
  line L586 (158.1888, -60.3767) -> (157.7825, -60.1036)
  line L587 (203.8403, -4.439) -> (203.7228, -4.386)
  line L588 (177.5091, -80.8102) -> (177.6055, -80.3294)
  line L589 (156.8122, -62.4253) -> (156.8122, -79.1663)
  line L590 (158.1884, -24.0399) -> (158.4597, -23.6331)
  line L591 (156.4053, -79.4399) -> (156.1339, -79.8483)
  line L592 (206.966, -5.2003) -> (204.5263, -5.2003)
  line L593 (157.7825, -24.3125) -> (158.1884, -24.0399)
  line L594 (177.5102, -42.6819) -> (177.6055, -42.2017)
  line L595 (139.4102, -60.7842) -> (139.1388, -60.3767)
  line L596 (208.5558, -5.0475) -> (208.5286, -4.7436)
  line L597 (191.4903, 0.081) -> (190.9024, -0.5069)
  line L598 (200.2376, -3.9348) -> (199.9607, -4.0327)
  line L599 (204.5057, -4.9107) -> (204.3632, -4.6576)
  line L600 (199.7531, -4.2406) -> (199.6558, -4.5177)
  line L601 (200.4629, -5.2764) -> (200.5471, -5.2842)
  line L602 (199.6877, -4.8097) -> (199.8426, -5.0593)
  line L603 (199.8426, -5.0593) -> (200.0901, -5.2175)
  line L604 (213.5483, -8.0034) -> (213.8751, -8.0076)
  line L605 (202.7938, -5.3116) -> (202.7599, -5.3424)
  line L606 (202.0993, -5.7801) -> (201.8671, -6.0134)
  line L607 (202.7599, -5.3424) -> (202.415, -5.6873)
  line L608 (200.0901, -5.2175) -> (200.3816, -5.2532)
  line L609 (204.3632, -4.6576) -> (204.1263, -4.4896)
  line L610 (214.3454, -7.5832) -> (214.3747, -7.2577)
  line L611 (200.5471, -5.2842) -> (202.8304, -5.2842)
  line L612 (200.9382, -4.3679) -> (200.7795, -4.1206)
  line L613 (202.8304, -5.2842) -> (202.7938, -5.3116)
  line L614 (208.3683, -4.4841) -> (208.1088, -4.3238)
  line L615 (213.9416, -5.8848) -> (213.6754, -5.7176)
  line L616 (200.3816, -5.2532) -> (200.4629, -5.2764)
  line L617 (200.5297, -3.9662) -> (200.2376, -3.9348)
  line L618 (203.1011, -6.3734) -> (203.3039, -6.1706)
  line L619 (203.3039, -6.1706) -> (207.1669, -6.1706)
  line L620 (204.5263, -5.2003) -> (204.5057, -4.9107)
  line L621 (212.8706, -6.0548) -> (212.803, -6.3619)
  line L622 (207.8049, -4.2966) -> (207.5211, -4.4084)
  line L623 (207.51, -6.0285) -> (207.9228, -5.6157)
  line L624 (201.8671, -6.0134) -> (201.7756, -6.3295)
  line L625 (62.5323, -79.1663) -> (62.5323, -62.4253)
  line L626 (120.3607, -79.8483) -> (120.0893, -79.4399)
  line L627 (137.3552, -79.4399) -> (137.0838, -79.8483)
  line L628 (63.3053, -61.2644) -> (63.21, -60.7842)
  line L629 (62.9392, -79.4399) -> (62.5323, -79.1663)
  line L630 (120.4554, -80.3294) -> (120.3607, -79.8483)
  line L631 (118.0341, -23.6313) -> (118.3055, -24.0392)
  line L632 (42.5119, -62.4253) -> (42.5119, -79.1663)
  line L633 (120.0893, -79.4399) -> (119.6824, -79.1663)
  line L634 (81.5823, -60.1036) -> (81.5823, -43.3625)
  line L635 (82.26, -60.7842) -> (81.9887, -60.3767)
  line L636 (81.9887, -60.3767) -> (81.5823, -60.1036)
  line L637 (137.0849, -22.6702) -> (136.9891, -23.1507)
  line L638 (100.6323, -43.3625) -> (101.0387, -43.0894)
  line L639 (101.0387, -43.0894) -> (101.3101, -42.6819)
  line L640 (145.1808, -15.532) -> (138.7251, -21.9878)
  line L641 (43.4822, -24.3125) -> (43.8881, -24.0399)
  line L642 (82.3553, -61.2644) -> (82.26, -60.7842)
  line L643 (81.9887, -62.1522) -> (82.26, -61.7447)
  line L644 (82.26, -61.7447) -> (82.3553, -61.2644)
  line L645 (81.9892, -79.4399) -> (81.5823, -79.1663)
  line L646 (81.5823, -79.1663) -> (81.5823, -62.4253)
  line L647 (61.5638, -21.99) -> (61.1568, -22.2627)
  line L648 (120.4554, -42.2017) -> (120.3601, -41.7214)
  line L649 (101.0387, -41.3139) -> (100.6323, -41.0408)
  line L650 (101.4053, -42.2017) -> (101.3101, -41.7214)
  line L651 (44.1595, -23.6331) -> (44.2552, -23.1536)
  line L652 (137.0838, -79.8483) -> (136.9891, -80.3294)
  line L653 (62.5323, -41.0408) -> (62.5323, -24.3125)
  line L654 (79.9343, -42.6819) -> (80.2056, -43.0894)
  line L655 (79.839, -42.2017) -> (79.9343, -42.6819)
  line L656 (101.3096, -23.6331) -> (101.4053, -23.1536)
  line L657 (42.1082, -81.2176) -> (42.5161, -81.4897)
  line L658 (63.3053, -80.3294) -> (63.2106, -79.8483)
  line L659 (137.3558, -43.0894) -> (137.7621, -43.3625)
  line L660 (62.5323, -62.4253) -> (62.9386, -62.1522)
  line L661 (61.1556, -43.0894) -> (61.562, -43.3625)
  line L662 (101.4053, -23.1536) -> (101.3111, -22.6739)
  line L663 (89.6875, -20.9069) -> (89.3974, -20.7906)
  line L664 (89.8921, -21.1432) -> (89.6875, -20.9069)
  line L665 (109.1488, -14.8362) -> (126.8266, -14.8362)
  line L666 (82.3553, -42.2017) -> (82.26, -41.7214)
  line L667 (82.26, -41.7214) -> (81.9887, -41.3139)
  line L668 (62.5249, -21.9878) -> (62.0441, -21.8935)
  line L669 (139.409, -80.8102) -> (139.5054, -80.3294)
  line L670 (88.8232, -20.9888) -> (83.9461, -20.9888)
  line L671 (120.0888, -41.3139) -> (119.6824, -41.0408)
  line L672 (89.3974, -20.7906) -> (89.0863, -20.8201)
  line L673 (63.21, -60.7842) -> (62.9386, -60.3767)
  line L674 (118.7121, -24.3125) -> (118.7121, -41.0408)
  line L675 (120.0861, -81.2176) -> (120.359, -80.8102)
  line L676 (81.9882, -24.0399) -> (82.2595, -23.6331)
  line L677 (81.5823, -41.0408) -> (81.5823, -24.3125)
  line L678 (81.5823, -24.3125) -> (81.9882, -24.0399)
  line L679 (118.3055, -24.0392) -> (118.7121, -24.3125)
  line L680 (118.7121, -41.0408) -> (118.3057, -41.3139)
  line L681 (80.2056, -43.0894) -> (80.612, -43.3625)
  line L682 (61.1554, -24.0392) -> (61.562, -24.3125)
  line L683 (137.7663, -81.4897) -> (138.2473, -81.5853)
  line L684 (80.2056, -41.3139) -> (79.9343, -41.7214)
  line L685 (98.8891, -23.1507) -> (98.9841, -23.6313)
  line L686 (63.2088, -80.8102) -> (63.3053, -80.3294)
  line L687 (42.105, -79.4399) -> (41.8336, -79.8483)
  line L688 (137.3558, -41.3139) -> (137.0844, -41.7214)
  line L689 (62.5281, -81.4897) -> (62.936, -81.2176)
  line L690 (137.7621, -62.4253) -> (137.7621, -79.1663)
  line L691 (41.8342, -61.7447) -> (42.1056, -62.1522)
  line L692 (99.2569, -22.2627) -> (98.9848, -22.6702)
  line L693 (98.9848, -22.6702) -> (98.8891, -23.1507)
  line L694 (119.6824, -24.3125) -> (120.0883, -24.0399)
  line L695 (43.8881, -24.0399) -> (44.1595, -23.6331)
  line L696 (61.1568, -22.2627) -> (60.8848, -22.6702)
  line L697 (62.9386, -43.0894) -> (63.21, -42.6819)
  line L698 (82.2589, -80.8102) -> (82.3553, -80.3294)
  line L699 (62.5323, -43.3625) -> (62.9386, -43.0894)
  line L700 (81.986, -81.2176) -> (82.2589, -80.8102)
  line L701 (81.0972, -81.5853) -> (81.5781, -81.4897)
  line L702 (81.5781, -81.4897) -> (81.986, -81.2176)
  line L703 (99.6621, -24.3125) -> (99.6621, -41.0408)
  line L704 (99.2557, -43.0894) -> (99.6621, -43.3625)
  line L705 (98.9841, -23.6313) -> (99.2555, -24.0392)
  line L706 (98.8891, -42.2017) -> (98.9843, -42.6819)
  line L707 (118.7121, -43.3625) -> (118.7121, -60.1036)
  line L708 (119.6782, -81.4897) -> (120.0861, -81.2176)
  line L709 (80.612, -79.1663) -> (80.2051, -79.4399)
  line L710 (80.2056, -62.1522) -> (80.612, -62.4253)
  line L711 (80.612, -62.4253) -> (80.612, -79.1663)
  line L712 (62.0441, -21.8935) -> (61.5638, -21.99)
  line L713 (136.9891, -23.1507) -> (137.0841, -23.6313)
  line L714 (43.8886, -43.0894) -> (44.16, -42.6819)
  line L715 (80.612, -41.0408) -> (80.2056, -41.3139)
  line L716 (60.8842, -41.7214) -> (60.789, -42.2017)
  line L717 (79.9343, -41.7214) -> (79.839, -42.2017)
  line L718 (118.3057, -62.1522) -> (118.7121, -62.4253)
  line L719 (89.0863, -20.8201) -> (88.8232, -20.9888)
  line L720 (63.2106, -79.8483) -> (62.9392, -79.4399)
  line L721 (41.7389, -80.3294) -> (41.8354, -80.8102)
  line L722 (62.0471, -81.5853) -> (62.5281, -81.4897)
  line L723 (43.4822, -79.1663) -> (43.4822, -62.4253)
  line L724 (120.359, -80.8102) -> (120.4554, -80.3294)
  line L725 (118.0344, -60.7842) -> (117.9391, -61.2644)
  line L726 (42.1056, -62.1522) -> (42.5119, -62.4253)
  line L727 (79.839, -80.3294) -> (79.9354, -80.8102)
  line L728 (80.2051, -79.4399) -> (79.9337, -79.8483)
  line L729 (79.9337, -79.8483) -> (79.839, -80.3294)
  line L730 (138.7282, -81.4897) -> (139.1361, -81.2176)
  line L731 (118.3057, -43.0894) -> (118.7121, -43.3625)
  line L732 (118.0344, -42.6819) -> (118.3057, -43.0894)
  line L733 (43.8886, -41.3139) -> (43.4822, -41.0408)
  line L734 (120.4554, -23.1536) -> (120.3611, -22.6739)
  line L735 (83.9461, -20.9888) -> (90.7337, -14.2012)
  line L736 (108.4116, -14.2012) -> (100.625, -21.9878)
  line L737 (89.0863, -22.0738) -> (89.3974, -22.1032)
  line L738 (83.0298, -21.9051) -> (88.8232, -21.9051)
  line L739 (88.8232, -21.9051) -> (89.0863, -22.0738)
  line L740 (60.789, -23.1507) -> (60.884, -23.6313)
  line L741 (82.2611, -22.6739) -> (83.0298, -21.9051)
  line L742 (82.2595, -23.6331) -> (82.3553, -23.1536)
  line L743 (82.3553, -23.1536) -> (82.2611, -22.6739)
  line L744 (90.7337, -14.2012) -> (108.4116, -14.2012)
  line L745 (44.2552, -23.1536) -> (44.161, -22.6739)
  line L746 (98.9843, -41.7214) -> (98.8891, -42.2017)
  line L747 (80.2054, -24.0392) -> (80.612, -24.3125)
  line L748 (80.612, -24.3125) -> (80.612, -41.0408)
  line L749 (137.7621, -41.0408) -> (137.3558, -41.3139)
  line L750 (79.934, -23.6313) -> (80.2054, -24.0392)
  line L751 (127.5638, -15.4712) -> (145.2551, -15.4712)
  line L752 (61.1583, -81.2176) -> (61.5662, -81.4897)
  line L753 (62.936, -81.2176) -> (63.2088, -80.8102)
  line L754 (118.7163, -81.4897) -> (119.1972, -81.5853)
  line L755 (44.16, -60.7842) -> (43.8886, -60.3767)
  line L756 (138.2443, -21.8935) -> (137.764, -21.99)
  line L757 (44.1605, -79.8483) -> (43.8891, -79.4399)
  line L758 (137.3558, -62.1522) -> (137.7621, -62.4253)
  line L759 (80.6162, -81.4897) -> (81.0972, -81.5853)
  line L760 (79.9354, -80.8102) -> (80.2083, -81.2176)
  line L761 (80.2083, -81.2176) -> (80.6162, -81.4897)
  line L762 (118.3057, -60.3767) -> (118.0344, -60.7842)
  line L763 (118.7121, -60.1036) -> (118.3057, -60.3767)
  line L764 (99.6639, -21.99) -> (99.2569, -22.2627)
  line L765 (100.625, -21.9878) -> (100.1442, -21.8935)
  line L766 (43.4822, -41.0408) -> (43.4822, -24.3125)
  line L767 (100.1442, -21.8935) -> (99.6639, -21.99)
  line L768 (80.2056, -60.3767) -> (79.9343, -60.7842)
  line L769 (89.9658, -21.4469) -> (89.8921, -21.1432)
  line L770 (80.612, -60.1036) -> (80.2056, -60.3767)
  line L771 (89.8921, -21.7507) -> (89.9658, -21.4469)
  line L772 (89.3974, -22.1032) -> (89.6875, -21.9869)
  line L773 (89.6875, -21.9869) -> (89.8921, -21.7507)
  line L774 (139.4107, -79.8483) -> (139.1393, -79.4399)
  line L775 (120.0883, -24.0399) -> (120.3596, -23.6331)
  line L776 (60.789, -80.3294) -> (60.8854, -80.8102)
  line L777 (120.3596, -23.6331) -> (120.4554, -23.1536)
  line L778 (79.9348, -22.6702) -> (79.839, -23.1507)
  line L779 (62.9386, -41.3139) -> (62.5323, -41.0408)
  line L780 (137.0856, -80.8102) -> (137.3584, -81.2176)
  line L781 (79.839, -23.1507) -> (79.934, -23.6313)
  line L782 (117.9391, -80.3294) -> (118.0355, -80.8102)
  line L783 (118.3057, -41.3139) -> (118.0344, -41.7214)
  line L784 (118.0344, -41.7214) -> (117.9391, -42.2017)
  line L785 (44.2552, -80.3294) -> (44.1605, -79.8483)
  line L786 (79.9343, -61.7447) -> (80.2056, -62.1522)
  line L787 (79.9343, -60.7842) -> (79.839, -61.2644)
  line L788 (79.839, -61.2644) -> (79.9343, -61.7447)
  line L789 (117.9391, -42.2017) -> (118.0344, -42.6819)
  line L790 (60.884, -23.6313) -> (61.1554, -24.0392)
  line L791 (63.3053, -42.2017) -> (63.21, -41.7214)
  line L792 (80.612, -43.3625) -> (80.612, -60.1036)
  line L793 (120.0888, -43.0894) -> (120.3601, -42.6819)
  line L794 (126.8266, -14.8362) -> (119.675, -21.9878)
  line L795 (119.1972, -81.5853) -> (119.6782, -81.4897)
  line L796 (101.0392, -79.4399) -> (100.6323, -79.1663)
  line L797 (100.6323, -79.1663) -> (100.6323, -62.4253)
  line L798 (82.2606, -79.8483) -> (81.9892, -79.4399)
  line L799 (119.675, -21.9878) -> (119.1943, -21.8935)
  line L800 (63.21, -41.7214) -> (62.9386, -41.3139)
  line L801 (137.3584, -81.2176) -> (137.7663, -81.4897)
  line L802 (80.2068, -22.2627) -> (79.9348, -22.6702)
  line L803 (60.8848, -22.6702) -> (60.789, -23.1507)
  line L804 (118.0338, -79.8483) -> (117.9391, -80.3294)
  line L805 (120.3601, -61.7447) -> (120.4554, -61.2644)
  line L806 (120.4554, -61.2644) -> (120.3601, -60.7842)
  line L807 (43.8891, -79.4399) -> (43.4822, -79.1663)
  line L808 (136.9891, -61.2644) -> (137.0844, -61.7447)
  line L809 (98.9837, -79.8483) -> (98.8891, -80.3294)
  line L810 (120.3601, -42.6819) -> (120.4554, -42.2017)
  line L811 (99.6663, -81.4897) -> (100.1472, -81.5853)
  line L812 (120.3601, -60.7842) -> (120.0888, -60.3767)
  line L813 (137.7621, -24.3125) -> (137.7621, -41.0408)
  line L814 (62.9386, -60.3767) -> (62.5323, -60.1036)
  line L815 (81.0942, -21.8935) -> (80.6139, -21.99)
  line L816 (81.575, -21.9878) -> (81.0942, -21.8935)
  line L817 (44.16, -61.7447) -> (44.2552, -61.2644)
  line L818 (60.8854, -80.8102) -> (61.1583, -81.2176)
  line L819 (137.0844, -41.7214) -> (136.9891, -42.2017)
  line L820 (61.562, -62.4253) -> (61.562, -79.1663)
  line L821 (61.1556, -41.3139) -> (60.8842, -41.7214)
  line L822 (43.8859, -81.2176) -> (44.1588, -80.8102)
  line L823 (61.5662, -81.4897) -> (62.0471, -81.5853)
  line L824 (137.0844, -60.7842) -> (136.9891, -61.2644)
  line L825 (136.9891, -80.3294) -> (137.0856, -80.8102)
  line L826 (44.16, -41.7214) -> (43.8886, -41.3139)
  line L827 (137.764, -21.99) -> (137.3569, -22.2627)
  line L828 (101.3101, -61.7447) -> (101.4053, -61.2644)
  line L829 (118.3084, -81.2176) -> (118.7163, -81.4897)
  line L830 (101.4053, -61.2644) -> (101.3101, -60.7842)
  line L831 (98.8891, -80.3294) -> (98.9855, -80.8102)
  line L832 (99.2552, -79.4399) -> (98.9837, -79.8483)
  line L833 (99.6621, -79.1663) -> (99.2552, -79.4399)
  line L834 (99.2557, -62.1522) -> (99.6621, -62.4253)
  line L835 (99.6621, -62.4253) -> (99.6621, -79.1663)
  line L836 (60.8837, -79.8483) -> (60.789, -80.3294)
  line L837 (61.1551, -79.4399) -> (60.8837, -79.8483)
  line L838 (43.4822, -43.3625) -> (43.8886, -43.0894)
  line L839 (120.3601, -41.7214) -> (120.0888, -41.3139)
  line L840 (61.562, -41.0408) -> (61.1556, -41.3139)
  line L841 (120.0888, -60.3767) -> (119.6824, -60.1036)
  line L842 (119.6824, -60.1036) -> (119.6824, -43.3625)
  line L843 (43.478, -81.4897) -> (43.8859, -81.2176)
  line L844 (137.0844, -61.7447) -> (137.3558, -62.1522)
  line L845 (101.3089, -80.8102) -> (101.4053, -80.3294)
  line L846 (101.4053, -80.3294) -> (101.3107, -79.8483)
  line L847 (139.1393, -79.4399) -> (138.7324, -79.1663)
  line L848 (100.6323, -62.4253) -> (101.0387, -62.1522)
  line L849 (119.6824, -43.3625) -> (120.0888, -43.0894)
  line L850 (80.6139, -21.99) -> (80.2068, -22.2627)
  line L851 (118.0355, -80.8102) -> (118.3084, -81.2176)
  line L852 (72.4457, -13.4392) -> (90.1235, -13.4392)
  line L853 (139.1361, -81.2176) -> (139.409, -80.8102)
  line L854 (63.211, -22.6739) -> (72.4457, -13.4392)
  line L855 (145.2165, -15.4997) -> (145.1808, -15.532)
  line L856 (61.1556, -62.1522) -> (61.562, -62.4253)
  line L857 (41.8354, -80.8102) -> (42.1082, -81.2176)
  line L858 (137.3555, -24.0392) -> (137.7621, -24.3125)
  line L859 (60.789, -61.2644) -> (60.8842, -61.7447)
  line L860 (61.562, -79.1663) -> (61.1551, -79.4399)
  line L861 (44.1588, -80.8102) -> (44.2552, -80.3294)
  line L862 (137.7621, -60.1036) -> (137.3558, -60.3767)
  line L863 (60.8842, -60.7842) -> (60.789, -61.2644)
  line L864 (60.789, -42.2017) -> (60.8842, -42.6819)
  line L865 (100.6323, -60.1036) -> (100.6323, -43.3625)
  line L866 (101.3101, -60.7842) -> (101.0387, -60.3767)
  line L867 (101.0387, -60.3767) -> (100.6323, -60.1036)
  line L868 (44.16, -42.6819) -> (44.2552, -42.2017)
  line L869 (100.1472, -81.5853) -> (100.6281, -81.4897)
  line L870 (100.6281, -81.4897) -> (101.036, -81.2176)
  line L871 (44.161, -22.6739) -> (54.1577, -12.6772)
  line L872 (101.3107, -79.8483) -> (101.0392, -79.4399)
  line L873 (98.9855, -80.8102) -> (99.2584, -81.2176)
  line L874 (99.2584, -81.2176) -> (99.6663, -81.4897)
  line L875 (101.036, -81.2176) -> (101.3089, -80.8102)
  line L876 (145.2551, -15.4712) -> (145.2165, -15.4997)
  line L877 (98.9843, -42.6819) -> (99.2557, -43.0894)
  line L878 (101.3101, -42.6819) -> (101.4053, -42.2017)
  line L879 (63.21, -61.7447) -> (63.3053, -61.2644)
  line L880 (119.1943, -21.8935) -> (118.7139, -21.99)
  line L881 (118.7139, -21.99) -> (118.3069, -22.2627)
  line L882 (42.5161, -81.4897) -> (42.9971, -81.5853)
  line L883 (137.7621, -43.3625) -> (137.7621, -60.1036)
  line L884 (101.0387, -62.1522) -> (101.3101, -61.7447)
  line L885 (82.3553, -80.3294) -> (82.2606, -79.8483)
  line L886 (81.5823, -62.4253) -> (81.9887, -62.1522)
  line L887 (118.3069, -22.2627) -> (118.0349, -22.6702)
  line L888 (43.8886, -62.1522) -> (44.16, -61.7447)
  line L889 (90.1235, -13.4392) -> (81.575, -21.9878)
  line L890 (63.2095, -23.6331) -> (63.3053, -23.1536)
  line L891 (61.562, -24.3125) -> (61.562, -41.0408)
  line L892 (62.9382, -24.0399) -> (63.2095, -23.6331)
  line L893 (101.3101, -41.7214) -> (101.0387, -41.3139)
  line L894 (61.562, -60.1036) -> (61.1556, -60.3767)
  line L895 (43.4822, -62.4253) -> (43.8886, -62.1522)
  line L896 (60.8842, -61.7447) -> (61.1556, -62.1522)
  line L897 (137.7621, -79.1663) -> (137.3552, -79.4399)
  line L898 (41.8336, -79.8483) -> (41.7389, -80.3294)
  line L899 (101.0382, -24.0399) -> (101.3096, -23.6331)
  line L900 (44.2552, -42.2017) -> (44.16, -41.7214)
  line L901 (100.6323, -24.3125) -> (101.0382, -24.0399)
  line L902 (100.6323, -41.0408) -> (100.6323, -24.3125)
  line L903 (54.1577, -12.6772) -> (71.8355, -12.6772)
  line L904 (139.5054, -80.3294) -> (139.4107, -79.8483)
  line L905 (82.26, -42.6819) -> (82.3553, -42.2017)